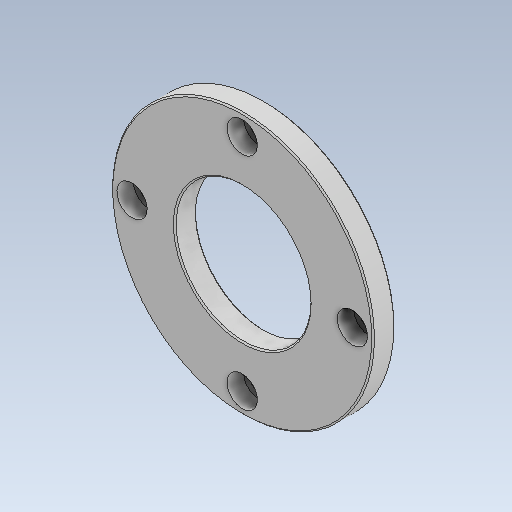
# Autodesk Inventor part: Peça22
Saved by Autodesk Inventor 2021 (Build 250183000, 183)
## iProperties
Category: 41
Created: 2021-07-19
Part Number: Peça22
Material: Genérico
Document SubType Name: Modeling
Designer: Giovanni
Density: 1 g/cm^3
Appearance: Padrão
User Status: 1:2
Author: Giovanni
Keywords: 28
Autodesk Inventor part; units mm, degrees
ref_plane "YZ Plane" through (0, 0, 0) normal (1, 0, 0) x (0, 1, 0)
ref_plane "XZ Plane" through (0, 0, 0) normal (0, 1, 0) x (-1, 0, 0)
ref_plane "XY Plane" through (0, 0, 0) normal (0, 0, 1) x (1, 0, 0)
sketch "Esboço1" plane through (0, 0, 0) normal (0, 0, 1) x (1, 0, 0)
  circle A0 centre (0, 0) radius 24.5
  circle A1 centre (0, 0) radius 47.5
  dimension "d0" = 49
  dimension "d1" = 95
  constraints: 2 centre point, 2 coincident
  measures "d0" diameter of A0
  measures "d1" diameter of A1
extrude "Extrusão1" add sketch "Esboço1" against normal blind 8
sketch "Esboço2" plane through (0, 0, -8) normal (0, 0, -1) x (-1, 0, 0)
  circle A0 centre (0, 0) radius 24.5 projected
  circle A1 centre (0, 0) radius 30
  circle A2 centre (0, 0) radius 34
  dimension "d4" = 60
  dimension "d5" = 68
  constraints: 2 centre point, 2 coincident
  measures "d4" diameter of A1
  measures "d5" diameter of A2
extrude "Extrusão2" add sketch "Esboço2" along normal blind 2 contours A2
sketch "Esboço3" plane through (0, 0, 0) normal (0, 0, 1) x (1, 0, 0)
  circle A0 centre (0, 0) radius 47.5 projected
  point P0 (0, 40)
  dimension "d8" = 40
  constraints: 1 vertical alignment
  measures "d8" distance of A0.centre point (0, 40)
hole "Furo1" at (0, 40, 0) direction (0, 0, -1) diameter 6.6 depth 10 tip angle 118 counterbore diameter 11 counterbore depth 6
pattern_circular "Padrão circular1" count 4 over 360 about axis through (0, 0, -10) along (0, 0, 1) of "Furo1"
chamfer "Chanfro1" distance 0.5 angle 45 6 edges at (-24.5, 0, 0) (-24.5, 0, -8) (-47.5, 0, 0) (-47.5, 0, -8) (34, 0, -10) (30, 0, -10)
